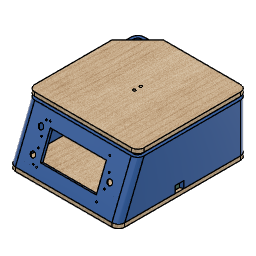
case (Autodesk Fusion 360 design; units mm, degrees)
Autodesk Fusion 360 part; units mm, degrees
ref_plane "WorkPlane2" through (0, 75, 0) normal (0, 1, 0) x (0, 0, 1)
sketch "Sketch1" plane through (0, 75, 0) normal (0, 1, 0) x (1, 0, 0)
  line L0 (75, -85) -> (-75, -85)
  line L1 (-85, -75) -> (-85, 75)
  line L2 (-75, 85) -> (75, 85)
  line L3 (85, 75) -> (85, -75)
  line L4 (85, -85) -> (-85, 85) construction
  line L5 (-85, -85) -> (85, 85) construction
  arc A0 (-75, 85) -> (-85, 75) centre (-75, 75) ccw
  arc A1 (85, 75) -> (75, 85) centre (75, 75) ccw
  arc A2 (75, -85) -> (85, -75) centre (75, -75) ccw
  arc A3 (-85, -75) -> (-75, -85) centre (-75, -75) ccw
  arc A4 (80.2, 75) -> (75, 80.2) centre (75, 75) ccw
  line L6 (-75, 80.2) -> (75, 80.2)
  arc A5 (-75, 80.2) -> (-80.2, 75) centre (-75, 75) ccw
  line L7 (-80.2, -75) -> (-80.2, 75)
  arc A6 (-80.2, -75) -> (-75, -80.2) centre (-75, -75) ccw
  line L8 (75, -80.2) -> (-75, -80.2)
  arc A7 (75, -80.2) -> (80.2, -75) centre (75, -75) ccw
  line L9 (80.2, 75) -> (80.2, -75)
  dimension "d1" = 170
  dimension "d3" = 10
  dimension "d6" = 4.8
  constraint horizontal L0
  constraint perpendicular L0 L1
  constraint parallel L0 L2
  constraint parallel L1 L3
  constraint coincident L4 origin
  constraint coincident L5 origin
  constraint coincident L4.end L2
  constraint coincident L4.end L1
  constraint tangent L2 A0
  constraint tangent L1 A0
  constraint coincident L5.end L2
  constraint coincident L5.end L3
  constraint tangent L2 A1
  constraint tangent L3 A1
  constraint equal A0 A1
  constraint coincident L4.start L3
  constraint coincident L4.start L0
  constraint tangent L3 A2
  constraint tangent L0 A2
  constraint coincident L5.start L1
  constraint coincident L5.start L0
  constraint tangent L1 A3
  constraint tangent L0 A3
  constraint equal A1 A2
  constraint equal A0 A3
  constraint equal L1 L2
  measures "d1" distance of L4.end L5.end
  measures "d3" radius of A0
sketch "Sketch2" plane through (0, 0, 0) normal (0, 1, 0) x (1, 0, 0)
  line L0 (-75, 85) -> (75, 85)
  line L1 (-85, 75) -> (-85, -105)
  line L2 (85, 75) -> (85, -105)
  line L3 (-75, -115) -> (75, -115)
  arc A0 (-75, 85) -> (-85, 75) centre (-75, 75) ccw
  arc A1 (85, 75) -> (75, 85) centre (75, 75) ccw
  arc A2 (-85, -105) -> (-75, -115) centre (-75, -105) ccw
  arc A3 (75, -115) -> (85, -105) centre (75, -105) ccw
  arc A4 (80.2, 75) -> (75, 80.2) centre (75, 75) ccw
  line L4 (-75, 80.2) -> (75, 80.2)
  arc A5 (-75, 80.2) -> (-80.2, 75) centre (-75, 75) ccw
  line L5 (-80.2, 75) -> (-80.2, -105)
  arc A6 (-80.2, -105) -> (-75, -110.2) centre (-75, -105) ccw
  line L6 (-75, -110.2) -> (75, -110.2)
  arc A7 (75, -110.2) -> (80.2, -105) centre (75, -105) ccw
  line L7 (80.2, 75) -> (80.2, -105)
  point P0 (-85, 85)
  point P1 (85, 85)
  point P2 (-85, -115)
  dimension "d7" = 170
  dimension "d8" = 85
  dimension "d9" = 85
  dimension "d10" = 200
  dimension "d11" = 10
  dimension "d15" = 4.8
  constraint horizontal L0
  constraint perpendicular L0 L1
  constraint perpendicular L0 L2
  constraint coincident P0 L0
  constraint coincident P0 L1
  constraint tangent L0 A0
  constraint tangent L1 A0
  constraint coincident P1 L0
  constraint coincident P1 L2
  constraint tangent L0 A1
  constraint tangent L2 A1
  constraint coincident P2 L1
  constraint coincident P2 L3
  constraint tangent L1 A2
  constraint tangent L3 A2
  constraint tangent L2 A3
  constraint tangent L3 A3
  constraint horizontal L3
  constraint equal A0 A2
  constraint equal A0 A1
  constraint equal A0 A3
  measures "d7" distance of P0 P1
  measures "d8" horizontal distance of P0 origin
  measures "d9" vertical distance of P0 origin
  measures "d10" distance of P0 P2
  measures "d11" radius of A0
loft "Loft1" add profiles "Sketch2", "Sketch1" section 1 section 2 makes body 1
loft "Loft2" cut profiles "Sketch1", "Sketch2" section 1 contours A4 L6 A5 L7 A6 L8 A7 L9 section 2 contours A4 L4 A5 L5 A6 L6 A7 L7 bodies 1
ref_plane "WorkPlane3" through (0, 62.3, 0) normal (0, 1, 0) x (0, 0, 1)
sketch "Sketch3" plane through (0, 62.3, 0) normal (0, 1, 0) x (1, 0, 0)
  circle A0 centre (0, 5) radius 2
  circle A1 centre (0, -5) radius 2
  circle A2 centre (0, 49) radius 2
  circle A3 centre (0, 59) radius 2
  line L0 (0, 0) -> (0, 40) construction
  line L1 (-6.35, 64.5) -> (6.35, 64.5)
  line L2 (-6.35, -10.5) -> (6.35, -10.5)
  line L3 (-6.35, 64.5) -> (-6.35, -10.5)
  line L4 (6.35, 64.5) -> (6.35, -10.5)
  dimension "d21" = 4
  dimension "d22" = 4
  dimension "d23" = 10
  dimension "d24" = 5
  dimension "d25" = 4
  dimension "d26" = 4
  dimension "d27" = 10
  dimension "d28" = 44
  dimension "d29" = 12.7
  dimension "d30" = 75
  dimension "d31" = 5.5
  dimension "d128" = 40
  constraint coincident L0.start origin
  constraint vertical L0
  constraint coincident A3.centre L0
  constraint coincident A2.centre L0
  constraint coincident A0.centre L0
  constraint coincident A1.centre L0
  constraint horizontal L1
  constraint symmetric L0 L1.start L1.end
  constraint horizontal L2
  constraint equal L1 L2
  constraint perpendicular L2 L3
  constraint coincident L2.start L3.end
  measures "d21" diameter of A0
  measures "d22" diameter of A1
  measures "d23" distance of A0.centre A1.centre
  measures "d24" distance of A0.centre L0.start
  measures "d25" diameter of A2
  measures "d26" diameter of A3
  measures "d27" distance of A2.centre A3.centre
  measures "d28" distance of A0.centre A2.centre
  measures "d29" distance of L1.start L1.end
  measures "d30" distance of L1.end L2.end
  measures "d31" vertical distance of A3.centre L1.start
  measures "d128" distance of L0.start L0.end
extrude "Extrude2" add sketch "Sketch3" along normal blind 12.7 separate body makes body 2
sketch "Sketch4" plane through (0, 39.6552, 99.1379) normal (0, 0.371391, 0.928477) x (1, 0, 0)
  line L0 (75, -42.7099) -> (75, 38.0675)
  line L1 (75, 38.0675) -> (-75, 38.0675)
  line L2 (-75, 38.0675) -> (-75, -42.7099)
  line L3 (-75, 38.0675) -> (75, 38.0675) construction
  line L4 (75, 38.0675) -> (75, -42.7099) construction
  line L5 (75, -42.7099) -> (-75, -42.7099) construction
  line L6 (-75, -42.7099) -> (-75, 38.0675) construction
  line L7 (43.5, 18.6788) -> (-43.5, 18.6788)
  line L8 (-43.5, 18.6788) -> (-43.5, -23.3212)
  line L9 (-43.5, -23.3212) -> (43.5, -23.3212)
  line L10 (43.5, -23.3212) -> (43.5, 18.6788)
  line L11 (43.5, 18.6788) -> (-43.5, -23.3212) construction
  line L12 (-43.5, 18.6788) -> (43.5, -23.3212) construction
  line L13 (0, -2.3212) -> (75, -2.3212) construction
  circle A0 centre (56.5, -2.3212) radius 4
  line L14 (-56.5, 14.6788) -> (-56.5, -19.3212) construction
  circle A1 centre (-56.5, -19.3212) radius 4
  circle A2 centre (-56.5, 14.6788) radius 4
  line L15 (-75, -42.7099) -> (75, 38.0675) construction
  line L16 (-75, 38.0675) -> (75, -42.7099) construction
  circle A3 centre (46.5, -30.3212) radius 1.25
  line L17 (46.5, -30.3212) -> (-46.5, -30.3212) construction
  line L18 (-46.5, -30.3212) -> (-46.5, 25.6788) construction
  line L19 (-46.5, 25.6788) -> (46.5, 25.6788) construction
  line L20 (46.5, 25.6788) -> (46.5, -30.3212) construction
  line L21 (46.5, -30.3212) -> (-46.5, 25.6788) construction
  line L22 (-46.5, -30.3212) -> (46.5, 25.6788) construction
  circle A4 centre (46.5, 25.6788) radius 1.25
  circle A5 centre (-46.5, 25.6788) radius 1.25
  circle A6 centre (-46.5, -30.3212) radius 1.25
  line L23 (-75, -42.7099) -> (75, -42.7099)
  point P0 (0, -2.3212)
  point P1 (0, -2.3212)
  point P2 (0, -2.3212)
  dimension "d38" = 87
  dimension "d39" = 42
  dimension "d42" = 8
  dimension "d43" = 13
  dimension "d52" = 8
  dimension "d53" = 8
  dimension "d54" = 13
  dimension "d58" = 34
  dimension "d76" = 3
  dimension "d77" = 7
  dimension "d78" = 2.5
  constraint coincident L0.start L4.end
  constraint coincident L1.end L2.start
  constraint horizontal L7
  constraint perpendicular L7 L8
  constraint parallel L7 L9
  constraint parallel L8 L10
  constraint coincident L11 P2
  constraint coincident L12 P2
  constraint coincident P2 P1
  constraint perpendicular L0 L13
  constraint coincident L13 A0.centre
  constraint parallel L6 L14
  constraint coincident L14.end A1.centre
  constraint coincident L14.start A2.centre
  constraint symmetric L13 L14.end L14.start
  constraint coincident L2.end L5.end
  constraint coincident L0.end L1.start
  constraint coincident P2 L16
  constraint coincident L4 L13.end
  constraint coincident P2 L15
  constraint horizontal L17
  constraint perpendicular L17 L18
  constraint parallel L17 L19
  constraint parallel L18 L20
  constraint coincident L21 P2
  constraint coincident L22 P2
  constraint coincident A3.centre L17.start
  constraint coincident L19.end L20.start
  constraint coincident L18.end L19.start
  constraint coincident L17.end L18.start
  constraint equal A3 A4
  constraint equal A4 A5
  constraint equal A5 A6
  measures "d38" distance of L8.end L9.end
  measures "d39" distance of L7.end L8.end
  measures "d42" diameter of A0
  measures "d43" horizontal distance of L7.start A0.centre
  measures "d52" diameter of A1
  measures "d53" diameter of A2
  measures "d54" horizontal distance of L7.end L14.end
  measures "d58" vertical distance of L14.start L14.end
  measures "d76" horizontal distance of L9.end A3.centre
  measures "d77" vertical distance of L9.end A3.centre
  measures "d78" diameter of A3
extrude "Extrude3" cut sketch "Sketch4" against normal blind 9 contours L7 L8 L9 L10 bodies 1
extrude "Extrude4" cut sketch "Sketch4" against normal blind 5 contours A0 | A1 | A2 bodies 1
extrude "Extrude9" cut sketch "Sketch4" against normal blind 10 contours A3 | A4 | A5 | A6 bodies 1
sketch "Sketch5" plane through (0, 38, 95) normal (0, -0.371391, -0.928477) x (-1, 0, 0)
  circle A0 centre (-56.5, -2.3212) radius 4
  line L0 (-43.5, 18.6788) -> (43.5, 18.6788)
  line L1 (43.5, 18.6788) -> (43.5, -23.3212)
  line L2 (43.5, -23.3212) -> (-43.5, -23.3212)
  line L3 (-43.5, -23.3212) -> (-43.5, 18.6788)
  line L4 (75, -40.9273) -> (75, 39.8502)
  line L5 (75, 39.8502) -> (-75, 39.8502)
  line L6 (-75, 39.8502) -> (-75, -40.9273)
  line L7 (-56.5, -2.3212) -> (-62, -2.3212) construction
  line L8 (-49, -15.3212) -> (-75, -15.3212)
  line L9 (-75, -15.3212) -> (-75, 10.6788)
  line L10 (-75, 10.6788) -> (-49, 10.6788)
  line L11 (-49, 10.6788) -> (-49, -15.3212)
  line L12 (-49, -15.3212) -> (-75, 10.6788) construction
  line L13 (-75, -15.3212) -> (-49, 10.6788) construction
  circle A1 centre (56.5, -19.3212) radius 4
  circle A2 centre (56.5, 14.6788) radius 4
  line L14 (49, 27.6788) -> (75, 27.6788)
  line L15 (75, 27.6788) -> (75, -32.3212)
  line L16 (75, -32.3212) -> (49, -32.3212)
  line L17 (49, -32.3212) -> (49, 27.6788)
  line L18 (49, 27.6788) -> (75, -32.3212) construction
  line L19 (75, 27.6788) -> (49, -32.3212) construction
  circle A3 centre (46.5, -30.3212) radius 1.25
  circle A4 centre (-46.5, -30.3212) radius 1.25
  circle A5 centre (46.5, 25.6788) radius 1.25
  circle A6 centre (-46.5, 25.6788) radius 1.25
  circle A7 centre (-46.5, -30.3212) radius 2.5
  circle A8 centre (46.5, -30.3212) radius 2.5
  circle A9 centre (46.5, 25.6788) radius 2.5
  circle A10 centre (-46.5, 25.6788) radius 2.5
  line L20 (-75, -40.9273) -> (75, -40.9273)
  line L21 (-52, 7.6788) -> (-52, -12.3212) construction
  line L22 (56.5, 14.6788) -> (61.5, 14.6788) construction
  line L23 (52, 24.6788) -> (52, 4.6788) construction
  line L24 (56.5, -19.3212) -> (61.5, -19.3212) construction
  line L25 (52, -9.3212) -> (52, -29.3212) construction
  line L26 (-49, 10.6788) -> (-52, 7.6788) construction
  line L27 (49, 27.6788) -> (52, 24.6788) construction
  line L28 (49, 27.6788) -> (52.5, 27.6788) construction
  line L29 (49, -32.3212) -> (52, -29.3212) construction
  line L30 (49, -32.3212) -> (52.5, -32.3212) construction
  circle A11 centre (52, 24.6788) radius 1.25
  circle A12 centre (52, 4.6788) radius 1.25
  circle A13 centre (52, -9.3212) radius 1.25
  circle A14 centre (52, -29.3212) radius 1.25
  circle A15 centre (-52, 7.6788) radius 1.25
  circle A16 centre (-52, -12.3212) radius 1.25
  circle A17 centre (52, 24.6788) radius 2.5
  circle A18 centre (52, -29.3212) radius 2.5
  circle A19 centre (52, -9.3212) radius 2.5
  circle A20 centre (52, 4.6788) radius 2.5
  circle A21 centre (-52, 7.6788) radius 2.5
  circle A22 centre (-52, -12.3212) radius 2.5
  circle A23 centre (-52, 7.6788) radius 1.65
  circle A24 centre (-52, -12.3212) radius 1.65
  circle A25 centre (52, 24.6788) radius 1.65
  circle A26 centre (52, 4.6788) radius 1.65
  circle A27 centre (52, -9.3212) radius 1.65
  circle A28 centre (52, -29.3212) radius 1.65
  line L31 (-62, -2.3212) -> (-62, 10.6788) construction
  line L32 (-66, 10.6788) -> (-66, 20.6788)
  line L33 (-66, 20.6788) -> (-58, 20.6788)
  line L34 (-58, 20.6788) -> (-58, 10.6788)
  line L35 (-66, -15.3212) -> (-66, -25.3212)
  line L36 (-66, -25.3212) -> (-58, -25.3212)
  line L37 (-58, -25.3212) -> (-58, -15.3212)
  line L38 (62, -2.3212) -> (62, 27.6788) construction
  line L39 (58, 27.6788) -> (58, 37.6788)
  line L40 (58, 37.6788) -> (66, 37.6788)
  line L41 (66, 37.6788) -> (66, 27.6788)
  line L42 (58, -32.3212) -> (58, -39.8212)
  line L43 (58, -39.8212) -> (66, -39.8212)
  line L44 (66, -39.8212) -> (66, -32.3212)
  point P0 (-62, -2.3212)
  point P1 (62, -2.3212)
  dimension "d46" = 26
  dimension "d47" = 7.5
  dimension "d55" = 26
  dimension "d57" = 7.5
  dimension "d59" = 13
  dimension "d60" = 13
  dimension "d81" = 5
  dimension "d104" = 5
  dimension "d105" = 5
  dimension "d106" = 45
  dimension "d107" = 45
  dimension "d108" = 3
  dimension "d109" = 3.5
  dimension "d110" = 3.5
  dimension "d111" = 2.5
  dimension "d112" = 5
  dimension "d113" = 3.3
  dimension "d122" = 8
  dimension "d123" = 10
  dimension "d124" = 7.5
  constraint coincident A0.centre L7.start
  constraint perpendicular L3 L7
  constraint horizontal L8
  constraint perpendicular L8 L9
  constraint parallel L8 L10
  constraint parallel L9 L11
  constraint coincident L12 P0
  constraint coincident L13 P0
  constraint coincident P0 L7.end
  constraint equal L9 L10
  constraint horizontal L14
  constraint perpendicular L14 L15
  constraint parallel L14 L16
  constraint parallel L15 L17
  constraint coincident L18 P1
  constraint coincident L19 P1
  constraint concentric A4 A7
  constraint concentric A3 A8
  constraint concentric A5 A9
  constraint concentric A6 A10
  constraint equal A8 A9
  constraint equal A7 A8
  constraint equal A7 A10
  constraint symmetric L7 L21.start L21.end
  constraint coincident A2.centre L22.start
  constraint perpendicular L17 L22
  constraint symmetric L22 L23.end L23.start
  constraint coincident A1.centre L24.start
  constraint horizontal L24
  constraint vertical L25
  constraint symmetric L24 L25.start L25.end
  constraint coincident L13 L21.start
  constraint coincident L21.start L26.end
  constraint horizontal L28
  constraint horizontal L30
  constraint coincident L25.end L29.end
  constraint equal L27 L29
  constraint equal L26 L27
  constraint coincident L23.start L27.end
  constraint coincident L23.end A12.centre
  constraint coincident L25.start A13.centre
  constraint coincident L21.end A16.centre
  constraint equal A14 A16
  constraint equal A13 A14
  constraint equal A11 A13
  constraint equal A11 A12
  constraint equal A12 A15
  constraint concentric A11 A17
  constraint concentric A13 A19
  constraint concentric A12 A20
  constraint concentric A15 A21
  constraint equal A17 A20
  constraint equal A19 A20
  constraint equal A18 A19
  constraint equal A18 A21
  constraint equal A21 A22
  constraint concentric A15 A23
  constraint concentric A16 A24
  constraint concentric A11 A25
  constraint concentric A20 A26
  constraint concentric A13 A27
  constraint concentric A14 A28
  constraint equal A23 A24
  constraint equal A24 A25
  constraint equal A25 A26
  constraint equal A26 A27
  constraint equal A27 A28
  constraint midpoint L10 L31.end
  constraint coincident L10 L32.start
  constraint perpendicular L10 L32
  constraint perpendicular L32 L33
  constraint coincident L10 L34.end
  constraint perpendicular L10 L34
  constraint symmetric L31 L32.start L34.end
  constraint coincident L8 L35.start
  constraint perpendicular L8 L35
  constraint perpendicular L35 L36
  constraint coincident L8 L37.end
  constraint perpendicular L8 L37
  constraint equal L34 L37
  constraint equal L33 L36
  constraint symmetric L31 L35.start L37.end
  constraint coincident P1 L38.start
  constraint midpoint L14 L38.end
  constraint coincident L14 L39.start
  constraint perpendicular L14 L39
  constraint perpendicular L39 L40
  constraint coincident L14 L41.end
  constraint perpendicular L14 L41
  constraint symmetric L38 L39.start L41.end
  constraint equal L34 L39
  constraint equal L33 L40
  constraint coincident L16 L42.start
  constraint perpendicular L16 L42
  constraint perpendicular L42 L43
  constraint coincident L16 L44.end
  constraint perpendicular L16 L44
  constraint symmetric L38 L42.start L44.end
  constraint equal L33 L43
  measures "d46" distance of L9.end L10.end
  measures "d47" horizontal distance of A0.centre L10.end
  measures "d55" distance of L15.end L16.end
  measures "d57" horizontal distance of A1.centre L16.end
  measures "d59" vertical distance of A1.centre L16.end
  measures "d60" vertical distance of A2.centre L14.start
  measures "d81" diameter of A7
  measures "d104" distance of A2.centre L22.end
  measures "d105" distance of A1.centre L24.end
  measures "d106" angle of L27 L28
  measures "d107" angle of L29 L30
  measures "d108" horizontal distance of L14.start L23.start
  measures "d109" distance of L16.end L30.end
  measures "d110" distance of L14.start L28.end
  measures "d111" diameter of A11
  measures "d112" diameter of A17
  measures "d113" diameter of A23
  measures "d122" distance of L32.end L33.end
  measures "d123" distance of L32.start L32.end
  measures "d124" distance of L42.start L42.end
extrude "Extrude5" cut sketch "Sketch5" along normal blind 4 and the other way blind 3 contours L4 L14 L15 L16 L17 | L16 L42 L43 L44 | L6 L8 L9 L10 L11 | L14 L39 L40 L41 | L8 L35 L36 L37 | L10 L32 L33 L34 | A11 | A12 | A13 | A14 | A15 | A16 | A17 | A18 | A19 | A20 | A21 | A22 | A23 | A24 | A25 | A26 | A27 | A28 bodies 1
sketch "Sketch6" plane through (0, 62.3, 0) normal (0, -1, 0) x (1, 0, 0)
  circle A0 centre (0, -5) radius 2
  circle A1 centre (0, 5) radius 2
  circle A2 centre (0, -49) radius 2
  circle A3 centre (0, -59) radius 2
  line L0 (-6.35, 10.5) -> (-6.35, -64.5)
  line L1 (-6.35, -64.5) -> (6.35, -64.5)
  line L2 (6.35, -64.5) -> (6.35, 10.5)
  line L3 (6.35, 10.5) -> (-6.35, 10.5)
  circle A4 centre (0, -59) radius 2
  circle A5 centre (0, -49) radius 2
  line L4 (-6.35, -43.5) -> (6.35, -43.5)
  line L5 (6.35, -43.5) -> (6.35, -64.5)
  line L6 (6.35, -64.5) -> (-6.35, -64.5)
  line L7 (-6.35, -64.5) -> (-6.35, -43.5)
  dimension "d61" = 4
  dimension "d62" = 4
  dimension "d64" = 5.5
  constraint horizontal L4
  constraint vertical L5
  constraint horizontal L6
  constraint vertical L7
  constraint coincident L2 L1.end
  constraint coincident A3.centre A4.centre
  constraint coincident A2.centre A5.centre
  constraint coincident L1.end L2.start
  constraint coincident L0.end L1.start
  measures "d61" diameter of A5
  measures "d62" diameter of A4
  measures "d64" vertical distance of A2.centre L4.end
sketch "Sketch7" plane through (80.2, 0, 0) normal (-1, 0, 0) x (0, 0, 1)
  line L0 (105, 0) -> (75, 75)
  line L1 (75, 75) -> (-75, 75)
  line L2 (-75, 75) -> (-75, 0)
  line L3 (8.4675, 0) -> (31.4675, 0)
  line L4 (31.4675, 0) -> (31.4675, 43)
  line L5 (31.4675, 43) -> (8.4675, 43)
  line L6 (8.4675, 43) -> (8.4675, 0)
  line L7 (24.9675, 0) -> (14.9675, 0)
  line L8 (14.9675, 0) -> (14.9675, 9)
  line L9 (14.9675, 9) -> (24.9675, 9)
  line L10 (24.9675, 9) -> (24.9675, 0)
  line L11 (24.9675, 0) -> (14.9675, 9) construction
  line L12 (14.9675, 0) -> (24.9675, 9) construction
  line L13 (14.9675, 0) -> (8.4675, 0) construction
  line L14 (24.9675, 0) -> (31.4675, 0) construction
  line L15 (-75, 0) -> (105, 0)
  point P0 (19.9675, 4.5)
  dimension "d67" = 43
  dimension "d68" = 23
  dimension "d69" = 4.5
  dimension "d70" = 9
  dimension "d71" = 10
  dimension "d127" = 83.4675
  constraint horizontal L3
  constraint vertical L4
  constraint horizontal L5
  constraint vertical L6
  constraint horizontal L7
  constraint perpendicular L7 L8
  constraint parallel L7 L9
  constraint parallel L8 L10
  constraint coincident L11 P0
  constraint coincident L12 P0
  constraint coincident L6 L3.start
  constraint perpendicular L6 L13
  constraint coincident L4 L3.end
  constraint perpendicular L4 L14
  constraint equal L13 L14
  constraint coincident L3.end L15
  measures "d67" distance of L3.end L4.end
  measures "d68" distance of L3.start L3.end
  measures "d69" vertical distance of L3.end P0
  measures "d70" distance of L7.end L8.end
  measures "d71" distance of L8.end L9.end
  measures "d127" distance of L2.end L3.start
extrude "Extrude7" add sketch "Sketch7" along normal blind 52 separate body contours L3 L4 L5 L6 L8 L9 L10 L15 | L3 L7 L8 L9 L10 L15 makes body 3
extrude "Extrude8" cut sketch "Sketch7" against normal blind 10 draft 20 contours L3 L7 L8 L9 L10 L15 bodies 1
extrude "Extrude10" add sketch "Sketch5" along normal blind 4 separate body contours A8 | A9 | A7 | A10 makes body 4 at (44.0124, 9.1212, 105.1155) makes body 5 at (44.0124, 61.1159, 84.3176) makes body 6 at (-48.9876, 9.1212, 105.1155) makes body 7 at (-48.9876, 61.1159, 84.3176)
sketch "Sketch8" plane through (0, 62.3, 0) normal (0, -1, 0) x (1, 0, 0)
  circle A0 centre (0, -59) radius 2
  circle A1 centre (0, -49) radius 2
  circle A2 centre (0, -5) radius 2
  circle A3 centre (0, 5) radius 2
  line L0 (-6.35, 10.5) -> (-6.35, -64.5)
  line L1 (-6.35, -64.5) -> (6.35, -64.5)
  line L2 (6.35, -64.5) -> (6.35, 10.5)
  line L3 (6.35, 10.5) -> (-6.35, 10.5)
  line L4 (18.25, -80) -> (-18.25, -80)
  line L5 (-18.25, -80) -> (-18.25, -43.5)
  line L6 (-18.25, -43.5) -> (18.25, -43.5)
  line L7 (18.25, -43.5) -> (18.25, -80)
  line L8 (0, -49) -> (0, -59) construction
  dimension "d88" = 36.5
  dimension "d89" = 5.5
  dimension "d90" = 36.5
  constraint horizontal L4
  constraint vertical L5
  constraint horizontal L6
  constraint vertical L7
  constraint coincident A1.centre L8.start
  constraint coincident A0.centre L8.end
  constraint symmetric L5.end L6.end L8
  measures "d88" distance of L4.end L5.end
  measures "d89" vertical distance of A1.centre L6.end
  measures "d90" distance of L5.end L6.end
extrude "Extrude12" add sketch "Sketch2" against normal blind 6 separate body contours L0 L1 L2 L3 A0 A1 A2 A3 | A4 L4 A5 L5 A6 L6 A7 L7 makes body 8
extrude "Extrude11" add sketch "Sketch8" along normal up to surface (62.3 mm away) separate body contours L0 L1 L2 L6 | L0 L1 L2 L4 L5 L6 L7 makes body 9
sketch "Sketch9" plane through (0, 75, 0) normal (0, 1, 0) x (-1, 0, 0)
  circle A0 centre (0, -59) radius 2
  circle A1 centre (0, -49) radius 2
  circle A2 centre (0, -5) radius 2
  circle A3 centre (0, 5) radius 2
  line L0 (6.35, -64.5) -> (6.35, 10.5)
  line L1 (6.35, 10.5) -> (-6.35, 10.5)
  line L2 (-6.35, 10.5) -> (-6.35, -64.5)
  line L3 (-6.35, -64.5) -> (6.35, -64.5)
  line L4 (-6.35, 10.5) -> (6.35, 10.5)
  line L5 (6.35, 10.5) -> (6.35, -10.5)
  line L6 (6.35, -10.5) -> (-6.35, -10.5)
  line L7 (-6.35, -10.5) -> (-6.35, 10.5)
  dimension "d91" = 5.5
  constraint horizontal L4
  constraint vertical L5
  constraint horizontal L6
  constraint vertical L7
  constraint coincident L0 L5.end
  constraint coincident L1.end L2.start
  measures "d91" vertical distance of A2.centre L5.end
extrude "Extrude13" add sketch "Sketch9" along normal blind 5 separate body contours L0 L1 L2 L4 L5 L6 L7 makes body 10
sketch "Sketch10" plane through (0, 80, 0) normal (0, 1, 0) x (-1, 0, 0)
  circle A0 centre (0, -5) radius 2
  circle A1 centre (0, 5) radius 2
  line L0 (-6.35, -10.5) -> (6.35, -10.5)
  line L1 (6.35, -10.5) -> (6.35, 10.5)
  line L2 (6.35, 10.5) -> (-6.35, 10.5)
  line L3 (-6.35, 10.5) -> (-6.35, -10.5)
  line L4 (75, 85) -> (-75, 85)
  line L5 (-85, 75) -> (-85, -75)
  line L6 (-75, -85) -> (45, -85)
  line L7 (85, -45) -> (85, 75)
  line L8 (85, 85) -> (-85, -85) construction
  line L9 (-85, 85) -> (85, -85) construction
  arc A2 (-85, -75) -> (-75, -85) centre (-75, -75) ccw
  arc A3 (-75, 85) -> (-85, 75) centre (-75, 75) ccw
  arc A4 (85, 75) -> (75, 85) centre (75, 75) ccw
  line L10 (85, -45) -> (45, -85)
  point P0 (85, -85)
  dimension "d94" = 170
  dimension "d95" = 170
  dimension "d101" = 40
  dimension "d102" = 40
  dimension "d103" = 10
  constraint horizontal L4
  constraint perpendicular L4 L5
  constraint parallel L4 L6
  constraint parallel L5 L7
  constraint coincident L8 origin
  constraint coincident L9 origin
  constraint coincident P0 L6
  constraint coincident P0 L7
  constraint coincident L8.end L6
  constraint coincident L8.end L5
  constraint tangent L6 A2
  constraint tangent L5 A2
  constraint coincident L9.start L5
  constraint coincident L9.start L4
  constraint tangent L5 A3
  constraint tangent L4 A3
  constraint coincident L8.start L7
  constraint coincident L8.start L4
  constraint tangent L7 A4
  constraint tangent L4 A4
  constraint equal A3 A4
  constraint equal A2 A3
  constraint coincident L7 P0
  constraint coincident L6 P0
  measures "d94" distance of L8.end P0
  measures "d95" distance of L9.start L8.end
  measures "d101" distance of L7.start P0
  measures "d102" distance of L6.end P0
  measures "d103" radius of A2
extrude "Extrude14" add sketch "Sketch10" along normal blind 6 separate body contours L0 L1 L2 L3 | L4 L5 L6 L7 A2 A3 A4 L10 makes body 11
extrude "Extrude15" add sketch "Sketch5" along normal blind 1 and the other way blind 3 separate body contours A17 | A18 | A19 | A20 | A21 | A22 | A23 | A24 | A25 | A26 | A27 | A28 makes body 12 at (-54.4969, 42.9712, 95.1656) makes body 13 at (49.5031, 45.7567, 94.0514) makes body 14 at (-54.4969, 29.9726, 100.365) makes body 15 at (-54.4969, 61.5408, 87.7378) makes body 16 at (49.5031, 27.1871, 101.4792) makes body 17 at (-54.4876, 10.9162, 106.9105)
extrude "Extrude16" add sketch "Sketch5" along normal blind 2.5 contours A23 | A24 | A25 | A26 | A27 | A28 bodies 12 13 14 15 16 17
extrude "Extrude17" cut sketch "Sketch5" against normal blind 6 contours A11 | A12 | A13 | A14 | A15 | A16 bodies 1
copy_body "Body->Comp1" bodies 1 removing the originals makes body 18 in component "Wall"
copy_body "Body->Comp2" bodies 8 removing the originals makes body 19 in component "Bottom plate"
copy_body "Body->Comp3" bodies 11 removing the originals makes body 20 in component "Top plate"
copy_body "Body->Comp4" bodies 9 removing the originals makes body 21 in component "Chunk of wood"
copy_body "Body->Comp5" bodies 10 removing the originals makes body 22 in component "Top plate spacer"
copy_body "Body->Comp6" bodies 2 removing the originals makes body 23 in component "Load cell"
copy_body "Body->Comp7" bodies 3 removing the originals makes body 24 in component "Microcontroller"
copy_body "Body->Comp8" bodies 4 removing the originals makes body 25 in component "LCD spacer 1"
copy_body "Body->Comp9" bodies 5 removing the originals makes body 26 in component "LCD spacer 2"
copy_body "Body->Comp10" bodies 7 removing the originals makes body 27 in component "LCD spacer 4"
copy_body "Body->Comp11" bodies 6 removing the originals makes body 28 in component "LCD spacer 3"
copy_body "Body->Comp12" bodies 12 removing the originals makes body 29 in component "Button spacer 1"
copy_body "Body->Comp13" bodies 17 removing the originals makes body 30 in component "Button spacer 6"
copy_body "Body->Comp14" bodies 13 removing the originals makes body 31 in component "Button spacer 2"
copy_body "Body->Comp15" bodies 15 removing the originals makes body 32 in component "Button spacer 4"
copy_body "Body->Comp16" bodies 14 removing the originals makes body 33 in component "Button spacer 3"
copy_body "Body->Comp17" bodies 16 removing the originals makes body 34 in component "Button spacer 5"
chamfer "Chamfer2" distance 3 angle 45 4 edges at (70.5, 47.915, 91.034) (53.5, 47.915, 91.034) (-53.5, 63.6991, 84.7203) (-70.5, 63.6991, 84.7203) on bodies 18 in component "Wall"
sketch "Sketch11" plane through (0, 0, 0) normal (0, -1, 0) x (1, 0, 0)
  line L0 (80.2, 8.4675) -> (80.2, 31.4675)
  line L1 (80.2, 31.4675) -> (28.2, 31.4675)
  line L2 (28.2, 31.4675) -> (28.2, 8.4675)
  line L3 (28.2, 8.4675) -> (80.2, 8.4675)
  line L4 (30.7, 28.9675) -> (77.2, 28.9675) construction
  line L5 (77.2, 28.9675) -> (77.2, 10.9675) construction
  line L6 (77.2, 10.9675) -> (30.7, 10.9675) construction
  line L7 (30.7, 10.9675) -> (30.7, 28.9675) construction
  circle A0 centre (30.7, 28.9675) radius 1.25
  circle A1 centre (30.7, 10.9675) radius 1.25
  circle A2 centre (77.2, 10.9675) radius 1.25
  circle A3 centre (77.2, 28.9675) radius 1.25
  dimension "d129" = 46.5
  dimension "d130" = 18
  dimension "d131" = 3
  dimension "d132" = 2.5
  dimension "d133" = 2.5
  constraint horizontal L4
  constraint vertical L5
  constraint horizontal L6
  constraint vertical L7
  constraint coincident L4.start L7.end
  constraint coincident L6.end L7.start
  constraint coincident L5.end L6.start
  constraint coincident L4.end L5.start
  constraint equal A0 A3
  constraint equal A2 A3
  constraint equal A1 A2
  measures "d129" distance of L4.start L4.end
  measures "d130" distance of L4.start L6.end
  measures "d131" horizontal distance of L0.end L4.end
  measures "d132" vertical distance of L0.end L4.end
  measures "d133" diameter of A0
extrude "Extrude1" cut sketch "Sketch11" along normal blind 6 contours A0 | A1 | A2 | A3 bodies 19 in component "Bottom plate"
component "Wall" placed x (1, 0, 0) y (0, 1, 0) z (0, 0, 1) at (0, 0, 0)
component "Bottom plate" placed x (1, 0, 0) y (0, 1, 0) z (0, 0, 1) at (0, 0, 0)
component "Top plate" placed x (1, 0, 0) y (0, 1, 0) z (0, 0, 1) at (0, 0, 0)
component "Chunk of wood" placed x (1, 0, 0) y (0, 1, 0) z (0, 0, 1) at (0, 0, 0)
component "Top plate spacer" placed x (1, 0, 0) y (0, 1, 0) z (0, 0, 1) at (0, 0, 0)
component "Load cell" placed x (1, 0, 0) y (0, 1, 0) z (0, 0, 1) at (0, 0, 0)
component "Microcontroller" placed x (1, 0, 0) y (0, 1, 0) z (0, 0, 1) at (0, 0, 0)
component "LCD spacer 1" placed x (1, 0, 0) y (0, 1, 0) z (0, 0, 1) at (0, 0, 0)
component "LCD spacer 2" placed x (1, 0, 0) y (0, 1, 0) z (0, 0, 1) at (0, 0, 0)
component "LCD spacer 4" placed x (1, 0, 0) y (0, 1, 0) z (0, 0, 1) at (0, 0, 0)
component "LCD spacer 3" placed x (1, 0, 0) y (0, 1, 0) z (0, 0, 1) at (0, 0, 0)
component "Button spacer 1" placed x (1, 0, 0) y (0, 1, 0) z (0, 0, 1) at (0, 0, 0)
component "Button spacer 6" placed x (1, 0, 0) y (0, 1, 0) z (0, 0, 1) at (0, 0, 0)
component "Button spacer 2" placed x (1, 0, 0) y (0, 1, 0) z (0, 0, 1) at (0, 0, 0)
component "Button spacer 4" placed x (1, 0, 0) y (0, 1, 0) z (0, 0, 1) at (0, 0, 0)
component "Button spacer 3" placed x (1, 0, 0) y (0, 1, 0) z (0, 0, 1) at (0, 0, 0)
component "Button spacer 5" placed x (1, 0, 0) y (0, 1, 0) z (0, 0, 1) at (0, 0, 0)
equation "d102 = d101"
named bodies: "Wall", "Load cell", "Microcontroller", "Bottom plate", "Chunk of wood", "Top plate spacer", "Top plate", "LCD spacer 1", "LCD spacer 2", "LCD spacer 3", "LCD spacer 4", "Button spacer 1", "Button spacer 2", "Button spacer 3", "Button spacer 4", "Button spacer 5", "Button spacer 6"
